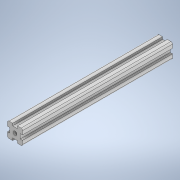
# Autodesk Inventor part: Profil
Saved by Autodesk Inventor 2021 (Build 250183000, 183)
## iProperties
Created: 2024-01-31
Part Number: Profil
Material: Generic
Document SubType Name: Modeling
Designer: Lukas
Density: 1 g/cm^3
Appearance: Default
Author: Lukas
Autodesk Inventor part; units mm, degrees
ref_plane "YZ Plane" through (0, 0, 0) normal (1, 0, 0) x (0, 1, 0)
ref_plane "XZ Plane" through (0, 0, 0) normal (0, 1, 0) x (-1, 0, 0)
ref_plane "XY Plane" through (0, 0, 0) normal (0, 0, 1) x (1, 0, 0)
sketch "Sketch1" plane through (0, 0, 0) normal (0, 0, 1) x (1, 0, 0)
  line L0 (-10, 10) -> (-3.15, 10)
  line L1 (-3.15, 10) -> (-3.15, 7)
  line L2 (-3.15, 7) -> (3.15, 7)
  line L3 (3.15, 7) -> (3.15, 10)
  line L4 (3.15, 10) -> (10, 10)
  line L5 (10, 10) -> (10, 3.15)
  line L6 (10, 3.15) -> (7, 3.15)
  line L7 (7, 3.15) -> (7, -3.15)
  line L8 (7, -3.15) -> (10, -3.15)
  line L9 (10, -3.15) -> (10, -10)
  line L10 (10, -10) -> (3.15, -10)
  line L11 (3.15, -10) -> (3.15, -7)
  line L12 (3.15, -7) -> (-3.15, -7)
  line L13 (-3.15, -7) -> (-3.15, -10)
  line L14 (-10, -10) -> (-10, -3.15)
  line L15 (-10, -3.15) -> (-7, -3.15)
  line L16 (-7, -3.15) -> (-7, 3.15)
  line L17 (-7, 3.15) -> (-10, 3.15)
  line L18 (-10, 10) -> (-10, 3.15)
  line L19 (-3.15, -10) -> (-10, -10)
  circle A0 centre (0, 0) radius 2.5
  point P0 (0, 7)
  point P1 (-7, 0)
  dimension "d0" = 20
  dimension "d1" = 6.3
  dimension "d2" = 3
  dimension "d3" = 5
  constraints: 40 end point, 19 perpendicular, 15 point on line, 2 midpoint, 1 centre point, 1 coincident, 1 horizontal, 1 horizontal alignment, 1 parallel, 1 vertical alignment
  measures "d0" distance between parallel lines of L5 L18
  measures "d1" distance between parallel lines of L15 L17
  measures "d2" distance of L16.end L17.end
  measures "d3" diameter of A0
extrude "Extrusion1" add sketch "Sketch1" along normal mid plane 200
fillet "Fillet1" radius 2 4 edges at (-10, 10, 0) (10, 10, 0) (10, -10, 0) (-10, -10, 0)
body "Solid1"
